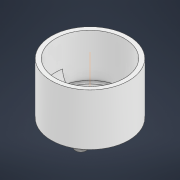
# Autodesk Inventor part: wheel
Saved by Autodesk Inventor 2022 (Build 260153000, 153)
## iProperties
Created: 2021-09-22
Part Number: wheel
Material: ABS プラスチック
Document SubType Name: Modeling
Designer: shiok
Density: 1.06 g/cm^3
Appearance: 滑らか - 白
Mass: 0.891598 g
Surface Area: 17.006 cm^2
Volume: 0.841131 cm^3
Author: shiok
Autodesk Inventor part; units mm, degrees
ref_plane "YZ Plane" through (0, 0, 0) normal (1, 0, 0) x (0, 1, 0)
ref_plane "XZ Plane" through (0, 0, 0) normal (0, 1, 0) x (-1, 0, 0)
ref_plane "XY Plane" through (0, 0, 0) normal (0, 0, 1) x (1, 0, 0)
sketch "スケッチ6" plane through (0, 0, 0) normal (0, 1, 0) x (-1, 0, 0)
  arc A0 (9, 0) -> (-4.5, 7.7942) centre (0, 0) ccw
  line L0 (0, 0) -> (-4.5, 7.7942) construction
  line L1 (0, 0) -> (9, 0) construction
  arc A1 (8, 0) -> (-4, 6.9282) centre (0, 0) ccw
  line L2 (0, 0) -> (-4, 6.9282) construction
  line L3 (0, 0) -> (8, 0) construction
  arc A2 (7, 0) -> (-3.5, 6.0622) centre (0, 0) ccw
  line L4 (0, 0) -> (-3.5, 6.0622) construction
  line L5 (0, 0) -> (7, 0) construction
  arc A3 (4.7, 0) -> (-2.35, 4.0703) centre (0, 0) ccw
  arc A4 (3.5, 0) -> (-1.75, 3.0311) centre (0, 0) ccw
  line L6 (4.5041, 1.3429) -> (6.7082, 2)
  arc A5 (10.9533, 0) -> (5.4767, 9.4859) centre (0, 0) ccw
  line L7 (0, 0) -> (5.4767, 9.4859) construction
  line L8 (0, 0) -> (10.9533, 0) construction
  line L9 (-1.0891, 4.5721) -> (-1.6221, 6.8095)
  line L10 (0, 0) -> (9, 0)
  line L11 (0, 0) -> (-4.5, 7.7942)
  point P0 (-1.6221, 6.8095)
  point P1 (-4, 6.9282)
  point P2 (-1.75, 3.0311)
  dimension "d33" = 9
  dimension "d34" = 120
  dimension "d35" = 120
  dimension "d36" = 1
  dimension "d37" = 120
  dimension "d38" = 2
  dimension "d39" = 4.7
  dimension "d40" = 3.5
  dimension "d41" = 2
  dimension "d42" = 60
  constraints: 24 end point, 14 point on circle, 6 centre point, 6 coincident, 5 point on line, 3 collinear, 2 midpoint, 2 symmetric about line, 1 horizontal
  measures "d33" radius of A0
  measures "d34" angle of L1 L0
  measures "d35" angle of L3 L2
  measures "d36" radial gap between concentric circles of A0 A1
  measures "d37" angle of L5 L4
  measures "d38" radial gap between concentric circles of A0 A2
  measures "d39" radius of A3
  measures "d40" radius of A4
  measures "d41" distance from line of L5 L6.end
  measures "d42" angle of L8 L7
extrude "押し出し6" add sketch "スケッチ6" along normal blind 1.9 contours L10 A2 L11 A1 | L10 A3 L6 A2 | A2 L9 A3 L11 | L10 A4 L11 A3
sketch "スケッチ7" plane through (0, 0, 0) normal (0, -1, 0) x (1, 0, 0)
  arc A0 (4, 6.9282) -> (-8, 0) centre (0, 0) ccw projected
  arc A1 (4.5, 7.7942) -> (-9, 0) centre (0, 0) ccw
  arc A2 (4, 6.9282) -> (-8, 0) centre (0, 0) ccw
  line L0 (0, 0) -> (4, 6.9282) construction
  line L1 (0, 0) -> (-8, 0) construction
  line L2 (4.5, 7.7942) -> (4, 6.9282)
  line L3 (-9, 0) -> (-8, 0)
  dimension "d45" = 120
  dimension "d46" = 9
  dimension "d47" = 8
  dimension "d48" = 120
  constraints: 8 end point, 4 point on circle, 2 centre point, 2 coincident, 1 horizontal
  measures "d46" radius of A1
  measures "d47" radius of A2
  measures "d48" angle of L0 L1
extrude "押し出し7" add sketch "スケッチ7" against normal blind 12
sketch "スケッチ8" plane through (0, 0, 0) normal (0, -1, 0) x (1, 0, 0)
  arc A0 (1.75, 3.0311) -> (-3.5, 0) centre (0, 0) ccw construction
  line L0 (-3.5, 0) -> (-8, 0) projected
  line L1 (0, 0) -> (-5.85, 0) construction
  arc A1 (-4.6, 0) -> (-7.1, 0) centre (-5.85, 0) ccw
  arc A2 (3.55, 6.1488) -> (2.3, 3.9837) centre (2.925, 5.0662) ccw
  line L2 (2.925, 5.0662) -> (2.3, 3.9837) construction
  line L3 (-5.85, 0) -> (-4.6, 0)
  line L4 (3.55, 6.1488) -> (1.75, 3.0311)
  line L5 (3.55, 6.1488) -> (2.3, 3.9837)
  line L6 (1.75, 3.0311) -> (4.5, 7.7942) projected
  line L7 (-7.9734, 0) -> (-7.1, 0)
  line L8 (-3.5, 0) -> (-9, 0) projected
  line L9 (4, 6.9282) -> (1.75, 3.0311) projected
  line L10 (4, 6.9282) -> (3.55, 6.1488)
  line L11 (1.0891, 4.5721) -> (1.6221, 6.8095) projected
  arc A3 (2.925, 5.0662) -> (-5.85, 0) centre (0, 0) ccw
  point P0 (-4.6, 0)
  dimension "d54" = 1.25
  dimension "d55" = 1.25
  dimension "d61" = 5.85
  constraints: 14 end point, 6 collinear, 6 point on circle, 5 point on line, 3 centre point, 3 coincident, 1 midpoint
  measures "d54" radius of A2
  measures "d55" radius of A1
  measures "d61" radius of A3
extrude "押し出し8" add sketch "スケッチ8" along normal blind 2
pattern_circular "円形状パターン1" count 3 over 360 about axis through (0, 0, 0) along (0, 1, 0)
sketch "スケッチ9" plane through (0, 0, 0) normal (0, -1, 0) x (1, 0, 0)
  circle A0 centre (0, 0) radius 4
  circle A1 centre (0, 0) radius 3.5 projected
  dimension "d62" = 8
  constraints: 1 centre point, 1 coincident
  measures "d62" diameter of A0
extrude "押し出し9" add sketch "スケッチ9" along normal up to surface (2 mm away)
sketch "スケッチ10" plane through (0, 1.9, 0) normal (0, 1, 0) x (1, 0, 0)
  arc A0 (-4.6178, 0.875) -> (-4.6178, -0.875) centre (0, 0) ccw
  line L0 (-4.6178, 0.875) -> (-7.8601, 1.4894)
  circle A1 centre (0, 0) radius 8 projected
  line L1 (-4.6178, -0.875) -> (-7.8601, -1.4894)
  line L2 (-4.7, 0) -> (-8, 0)
  line L3 (-8, 0) -> (-7.8601, 1.4894)
  line L4 (-8, 0) -> (-7.8601, -1.4894)
  dimension "d65" = 4.7
  dimension "d66" = 1.75
  constraints: 10 end point, 7 point on circle, 3 point on line, 1 centre point, 1 coincident, 1 equal length, 1 horizontal
  measures "d65" radius of A0
  measures "d66" distance of L1.start L0.start
extrude "押し出し10" add sketch "スケッチ10" along normal blind 3.3 contours A0 L2 L3 L0 | A0 L1 L4 L2 | L3 A1 | L4 A1
fillet "フィレット1" radius 3.3 1 edges at (-4.7, 5.2, 0) inverted yes
pattern_circular "円形状パターン2" count 3 over 360 about axis through (0, 0, 0) along (0, 1, 0) of "フィレット1", "押し出し10"
